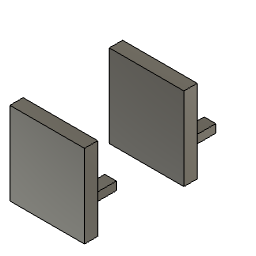
3d_3 (Autodesk Fusion 360 design; units mm, degrees)
Autodesk Fusion 360 part; units mm, degrees
box "BoxPrimitive1" add length 30 width 7 height 5 placed x (0, -1, 0) y (1, 0, 0) z (0, 0, 1) at (-20, 20, 0) makes body 1
box "BoxPrimitive2" add length 8 width 45 height 50 placed x (0, 1, 0) y (-1, 0, 0) z (0, 0, 1) at (-3.7154, -10.5425, 0) separate body makes body 2
move_body "Move1" bodies 2 to x (1, 0, 0) y (0, 1, 0) z (0, 0, 1) at (9, 0, 0)
sketch "Sketch3" plane through (0, 0, 0) normal (1, 0, 0) x (0, 1, 0)
sketch "Sketch4" plane through (0, 0, 0) normal (1, 0, 0) x (0, 1, 0)
  line L0 (4, 4) -> (-3, 10)
  line L1 (-3, 10) -> (-3, 4)
  line L2 (-3, 4) -> (4, 4)
  constraint vertical L1
  constraint perpendicular L1 L2
move_body "Move4" bodies 1 to x (1, 0, 0) y (0, 1, 0) z (0, 0, 1) at (0, 5, 0)
move_body "Move5" bodies 1 to x (1, 0, 0) y (0, 1, 0) z (0, 0, 1) at (0, 2, 0)
sketch "Sketch6" plane through (0, 0, 0) normal (1, 0, 0) x (0, 1, 0)
  line L0 (3, 4) -> (-4, 4)
  line L1 (-4, 4) -> (-4, 15)
  line L2 (-4, 15) -> (3, 4)
  constraint horizontal L0
  constraint perpendicular L0 L1
extrude "Extrude2" add sketch "Sketch6" along normal blind 7 separate body makes body 3
move_body "Move6" bodies 3 to x (1, 0, 0) y (0, 1, 0) z (0, 0, 1) at (-19, 0, 0)
move_body "Move7" bodies 3 to x (1, 0, 0) y (0, 1, 0) z (0, 0, 1) at (-1, 0, 0)
copy_body "CopyPasteBodies1" bodies 1 makes body 4
move_body "Move8" bodies 4 to x (1, 0, 0) y (0, 1, 0) z (0, 0, 1) at (0, 60, 0)
copy_body "CopyPasteBodies2" bodies 3 makes body 5
move_body "Move9" bodies 5 to x (1, 0, 0) y (0, 1, 0) z (0, 0, 1) at (0, 60, 0)
copy_body "CopyPasteBodies3" bodies 2 makes body 6
move_body "Move10" bodies 6 to x (1, 0, 0) y (0, 1, 0) z (0, 0, 1) at (0, 60, 0)
